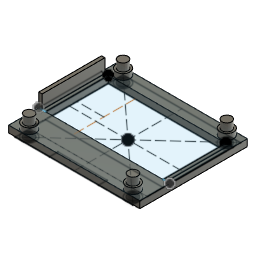
SH1106-LCD-Frame (Autodesk Fusion 360 design; units mm, degrees)
Autodesk Fusion 360 part; units mm, degrees
note: some values were not read from the file. Chosen so that the rebuilt part matches the saved one: which face or edge a step refers to.
sketch "Sketch1" plane through (0, 0, 0) normal (0, 1, 0) x (1, 0, 0)
  line L0 (17.2, 15.75) -> (-17.2, 15.75)
  line L1 (-17.2, 15.75) -> (-17.2, -15.75)
  line L2 (-17.2, -15.75) -> (17.2, -15.75)
  line L3 (17.2, -15.75) -> (17.2, 15.75)
  line L4 (17.2, 15.75) -> (-17.2, -15.75) construction
  line L5 (-17.2, 15.75) -> (17.2, -15.75) construction
  line L6 (17.2, 15.75) -> (15.2, 15.75) construction
  line L7 (15.2, 15.75) -> (15.2, 13.75) construction
  circle A0 centre (15.2, 13.75) radius 2
  circle A1 centre (15.2, 13.75) radius 1.425
  line L8 (0, -15.75) -> (0, 15.75) construction
  line L9 (-17.2, 0) -> (17.2, 0) construction
  circle A2 centre (-15.2, 13.75) radius 2
  circle A3 centre (-15.2, 13.75) radius 1.425
  circle A4 centre (-15.2, -13.75) radius 1.425
  circle A5 centre (-15.2, -13.75) radius 2
  circle A6 centre (15.2, -13.75) radius 1.425
  circle A7 centre (15.2, -13.75) radius 2
  line L10 (-17.2, -15.75) -> (-7.2, -15.75) construction
  line L11 (17.2, -15.75) -> (16.7785, -15.75) construction
  line L12 (17.2, -15.75) -> (7.2, -15.75) construction
  line L13 (7.2, -15.75) -> (7.2, -13.35)
  line L14 (7.2, -13.35) -> (-7.2, -13.35)
  line L15 (-7.2, -13.35) -> (-7.2, -15.75)
  line L16 (15.2, 13.75) -> (15.2, 11.75) construction
  line L17 (17.2, 11.45) -> (-17.4, 11.45)
  line L18 (-17.4, 11.45) -> (-17.4, -11.55) construction
  line L19 (-17.4, -11.55) -> (17.2, -11.55) construction
  line L20 (17.2, -11.55) -> (17.2, 11.45)
  line L21 (17.2, -11.55) -> (-17.2, -11.55) construction
  line L22 (-17.2, -11.55) -> (-17.2, -6.95) construction
  line L23 (-17.2, -6.95) -> (17.2, -6.95)
  line L24 (17.2, -6.95) -> (17.2, -11.55) construction
  line L25 (-9.3439, 11.45) -> (-9.3439, -6.95) construction
  line L26 (-9.3439, 2.25) -> (-17.2, 2.25) construction
  dimension "d1" = 34.4
  dimension "d2" = 31.5
  dimension "d4" = 2
  dimension "d5" = 2
  dimension "d6" = 4
  dimension "d7" = 2.85
  dimension "d8" = 10
  dimension "d9" = 10
  dimension "d10" = 2.4
  dimension "d11" = 34.6
  dimension "d12" = 23
  dimension "d13" = 4.6
  dimension "d14" = 0.3
  constraint horizontal L0
  constraint perpendicular L0 L1
  constraint parallel L0 L2
  constraint parallel L1 L3
  constraint coincident L4 origin
  constraint coincident L5 origin
  constraint perpendicular L3 L6
  constraint perpendicular L0 L7
  constraint coincident L7.end A0.centre
  constraint concentric A0 A1
  constraint midpoint L2 L8.start
  constraint midpoint L0 L8.end
  constraint midpoint L1 L9.start
  constraint midpoint L3 L9.end
  constraint symmetric A0 L8 A2
  constraint symmetric A1 L8 A3
  constraint symmetric A0 L9 A7
  constraint symmetric A1 L9 A6
  constraint symmetric L9 A2 A5
  constraint symmetric L9 A3 A4
  constraint perpendicular L1 L10
  constraint coincident L2 L11.end
  constraint perpendicular L3 L12
  constraint perpendicular L12 L13
  constraint perpendicular L13 L14
  constraint perpendicular L2 L15
  constraint coincident A0 L16.end
  constraint parallel L7 L16
  constraint coincident L3 L17.start
  constraint vertical L18
  constraint horizontal L19
  constraint vertical L20
  constraint horizontal L21
  constraint vertical L22
  constraint horizontal L23
  constraint vertical L24
  constraint coincident L1 L22.end
  constraint parallel L0 L17
  constraint coincident L17 L25.start
  constraint coincident L23 L25.end
  constraint perpendicular L23 L25
  constraint midpoint L25 L26.start
  constraint coincident L1 L26.end
  constraint perpendicular L1 L26
  measures "d1" distance of L1.end L2.end
  measures "d2" distance of L0.end L1.end
  measures "d4" distance of L0.start L6.end
  measures "d5" distance of L6.end L7.end
  measures "d6" diameter of A0
  measures "d7" diameter of A1
  measures "d8" distance of L1.end L10.end
  measures "d9" distance of L2.end L12.end
  measures "d10" distance of L12.end L13.end
  measures "d11" distance of L17.start L17.end
  measures "d12" distance of L17.start L19.end
  measures "d13" distance of L19.end L23.end
  measures "d14" distance of L16.end L17
extrude "Extrude1" add sketch "Sketch1" along normal blind 2
extrude "Extrude2" add 5 faces at (-17.2, 0.6667, -15.0833) (-17.2, 0.6667, -12.9833) (-17.2, 0.6667, -5.3167) (-17.2, 0.6667, 9.2167) (-17.2, 0.6667, 14.4167) along direction (-1, 0, 0) blind 2
move_face "OffsetFaces1" offset 2 1 faces at (17.2, 0.6667, 5.25)
extrude "Extrude3" cut sketch "Sketch1" along normal blind 3.756 contours L1 L3 L17 L20 L23
extrude "Extrude4" add sketch "Sketch1" along normal blind 3.72 contours A0 | A2 | A7 | A5
extrude "Extrude5" add sketch "Sketch1" along normal blind 6 contours A1 | A3 | A4 | A6
sketch "Sketch2" plane through (0, 2, 0) normal (0, 1, 0) x (-1, 0, 0)
  line L0 (17.2, 6.95) -> (17.2, -11.45)
  line L1 (17.2, -11.45) -> (-17.2, -11.45)
  line L2 (-17.2, -11.45) -> (-17.2, 6.95)
  line L3 (-17.2, 6.95) -> (17.2, 6.95)
  line L4 (-19.2, 15.75) -> (-19.2, -15.75)
  line L5 (-19.2, -15.75) -> (-15.2, -15.75)
  circle A0 centre (-15.2, -13.75) radius 2
  line L6 (-15.2, -15.75) -> (15.2, -15.75)
  circle A1 centre (15.2, -13.75) radius 2
  line L7 (15.2, -15.75) -> (19.2, -15.75)
  line L8 (19.2, -15.75) -> (19.2, 15.75)
  line L9 (19.2, 15.75) -> (15.2, 15.75)
  circle A2 centre (15.2, 13.75) radius 2
  line L10 (15.2, 15.75) -> (-15.2, 15.75)
  circle A3 centre (-15.2, 13.75) radius 2
  line L11 (-15.2, 15.75) -> (-19.2, 15.75)
  line L12 (17.2, -11.45) -> (19.2, -11.45)
  line L13 (19.2, -11.45) -> (19.2, 6.95)
  line L14 (19.2, 6.95) -> (17.2, 6.95)
  line L15 (17.2, 6.95) -> (17.2, -11.45)
  line L16 (-17.2, -11.45) -> (-19.2, -11.45)
  line L17 (-19.2, -11.45) -> (-19.2, 6.95)
  line L18 (-19.2, 6.95) -> (-17.2, 6.95)
  line L19 (-17.2, 6.95) -> (-17.2, -11.45)
  line L20 (18.2, -11.45) -> (18.2, 6.95)
  line L21 (-18.2, -11.45) -> (-18.2, 6.95)
  constraint horizontal L12
  constraint vertical L13
  constraint horizontal L14
  constraint vertical L15
  constraint coincident L8 L13.end
  constraint coincident L0.end L1.start
  constraint horizontal L16
  constraint vertical L17
  constraint horizontal L18
  constraint vertical L19
  constraint coincident L4 L17.end
  constraint coincident L1.end L2.start
  constraint midpoint L12 L20.start
  constraint midpoint L14 L20.end
  constraint midpoint L16 L21.start
  constraint midpoint L18 L21.end
extrude "Extrude9" add sketch "Sketch2" along normal blind 4 contours L8 L12 L13 L14 L20
extrude "Extrude6" [rolled back] along distance 4.1 taper angle 0
sketch "Sketch3" plane through (0, 6.1, 0) normal (0, 1, 0) x (-1, 0, 0)
  line L0 (18.2, -11.45) -> (18.2, 6.95)
  line L1 (18.2, 6.95) -> (17.2, 6.95)
  line L2 (17.2, 6.95) -> (17.2, -11.45)
  line L3 (17.2, -11.45) -> (18.2, -11.45)
  line L4 (17.2, -2.25) -> (18.2, -2.25) construction
  line L5 (17.2, 0.25) -> (18.2, 0.25)
  line L6 (18.2, 0.25) -> (18.2, -4.75) construction
  line L7 (18.2, -4.75) -> (17.2, -4.75)
  line L8 (17.2, -4.75) -> (17.2, 0.25) construction
  line L9 (17.2, 0.25) -> (18.2, -4.75) construction
  line L10 (18.2, 0.25) -> (17.2, -4.75) construction
  line L11 (0, 15.75) -> (0, -15.75) construction
  line L12 (-18.2, -4.75) -> (-17.2, -4.75)
  line L13 (-18.2, 0.25) -> (-18.2, -4.75) construction
  line L14 (-17.2, -4.75) -> (-17.2, 0.25) construction
  line L15 (-17.2, 0.25) -> (-18.2, 0.25)
  line L16 (-17.2, -4.75) -> (-18.2, -4.75)
  line L17 (-18.2, -4.75) -> (-18.2, 0.25)
  line L18 (-18.2, 0.25) -> (-17.2, 0.25)
  line L19 (-17.2, 0.25) -> (-17.2, -4.75)
  line L20 (17.2, -4.75) -> (16.7, -4.75)
  line L21 (16.7, -4.75) -> (16.7, 0.25)
  line L22 (16.7, 0.25) -> (17.2, 0.25)
  line L23 (17.2, 0.25) -> (17.2, -4.75)
  line L24 (-17.2, -4.75) -> (-16.7, -4.75)
  line L25 (-16.7, -4.75) -> (-16.7, 0.25)
  line L26 (-16.7, 0.25) -> (-17.2, 0.25)
  line L27 (-17.2, 0.25) -> (-17.2, -4.75)
  point P0 (17.7, -2.25)
  dimension "d28" = 5
  dimension "d29" = 0.5
  dimension "d30" = 0.5
  constraint midpoint L2 L4.start
  constraint midpoint L0 L4.end
  constraint horizontal L5
  constraint perpendicular L5 L6
  constraint parallel L5 L7
  constraint parallel L6 L8
  constraint coincident L9 P0
  constraint coincident L10 P0
  constraint midpoint L4 P0
  constraint symmetric L5.start L11 L14.end
  constraint symmetric L5.end L11 L13.start
  constraint symmetric L6.end L11 L12.start
  constraint symmetric L7.end L11 L12.end
  constraint horizontal L16
  constraint vertical L17
  constraint horizontal L18
  constraint vertical L19
  constraint horizontal L20
  constraint vertical L21
  constraint horizontal L22
  constraint vertical L23
  constraint horizontal L24
  constraint vertical L25
  constraint horizontal L26
  constraint vertical L27
  measures "d28" distance of L5.end L6.end
  measures "d29" distance of L7.end L20.end
  measures "d30" distance of L12.end L24.end
extrude "Extrude7" [rolled back] along distance 0.8 taper angle 0
extrude "Extrude8" [rolled back] along distance 0.8 taper angle 0
fillet "Fillet1" [rolled back] radius 0.5
chamfer "Chamfer1" [rolled back] distance 0.3
fillet "Fillet2" [rolled back] radius 0.5
chamfer "Chamfer2" [rolled back] distance 0.3
fillet "Fillet3" [rolled back] radius 0.5
equation "d22 = 2.00 mm + 1.72 mm"
